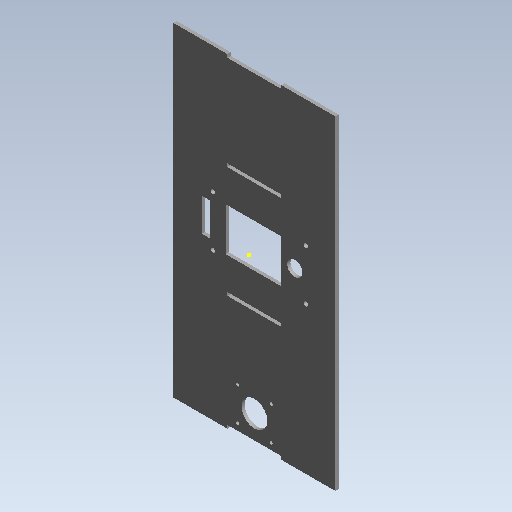
# Autodesk Inventor part: MuurL
Saved by Autodesk Inventor 2020 (Build 240168000, 168)
## iProperties
Part Number: MuurL
Material: Generic
Document SubType Name: Modeling
Designer: SBBA
Appearance: Default
Mass: 124.389 g
Surface Area: 879.905 cm^2
Volume: 124.389 cm^3
Density: 1 g/cm^3
Author: SBBA
Autodesk Inventor part; units mm, degrees
ref_plane "YZ Plane" through (0, 0, 0) normal (1, 0, 0) x (0, 1, 0)
ref_plane "XZ Plane" through (0, 0, 0) normal (0, 1, 0) x (-1, 0, 0)
ref_plane "XY Plane" through (0, 0, 0) normal (0, 0, 1) x (1, 0, 0)
sketch "Sketch1" plane through (0, 0, 0) normal (0, 0, 1) x (1, 0, 0)
  line L0 (-70.3712, 150.7033) -> (79.6288, 150.7033)
  line L1 (79.6288, 150.7033) -> (79.6288, -149.2967)
  line L2 (79.6288, -149.2967) -> (-70.3712, -149.2967)
  line L3 (-70.3712, -149.2967) -> (-70.3712, 150.7033)
  point P0 (0, 0)
  constraints: 8 end point, 2 parallel, 1 horizontal, 1 perpendicular
extrude "Extrusion1" add sketch "Sketch1" along normal blind 3
sketch "Sketch2" plane through (0, 0, 3) normal (0, 0, 1) x (1, 0, 0)
  line L0 (-70.3712, 150.7033) -> (-70.3712, -149.2967) projected
  line L1 (-70.3712, 271.0495) -> (-120.3712, 271.0495)
  line L2 (-20.3712, 147.7184) -> (-20.3712, 150.7184)
  line L3 (-20.3712, 147.7184) -> (29.6288, 147.7184)
  line L4 (29.6288, 147.7184) -> (29.6288, 150.7184)
  line L5 (-20.3712, 150.7184) -> (29.6288, 150.7184)
  line L6 (79.6288, 150.7033) -> (-70.3712, 150.7033) projected
  point P0 (0, 0)
  dimension "d9" = 50
  constraints: 10 end point, 2 horizontal, 2 vertical, 1 parallel, 1 point on line
  measures "d9" distance of L1.start L1.end
extrude "Extrusion2" cut sketch "Sketch2" against normal blind 3
sketch "Sketch3" plane through (0, 0, 3) normal (0, 0, 1) x (1, 0, 0)
  line L0 (-20.3712, 150.7033) -> (-20.3712, 147.7184) projected
  line L1 (-20.3712, -149.2722) -> (29.6288, -149.2967)
  line L2 (79.6288, -149.2967) -> (-70.3712, -149.2967) projected
  line L3 (-20.3712, -149.2722) -> (-20.3712, -146.2722)
  line L4 (-20.3712, -146.2722) -> (29.6288, -146.2967)
  line L5 (29.6288, -146.2967) -> (29.6288, -149.2967)
  point P0 (0, 0)
  constraints: 8 end point, 1 point on line, 1 vertical
extrude "Extrusion3" cut sketch "Sketch3" against normal blind 3
sketch "Sketch4" plane through (0, 0, 3) normal (0, 0, 1) x (1, 0, 0)
  line L0 (29.6288, -46.2722) -> (-20.3712, -46.2722)
  line L1 (-20.3712, -46.2722) -> (29.6288, -46.2722)
  line L2 (29.6288, -46.2722) -> (29.6288, -43.6172)
  line L3 (29.6288, -43.6172) -> (-20.3712, -43.6172)
  line L4 (-20.3712, -43.6172) -> (-20.3712, -46.2722)
  point P0 (0, 0)
  constraints: 10 end point, 2 parallel, 1 horizontal, 1 perpendicular
extrude "Extrusion4" add sketch "Sketch4" against normal blind 3
sketch "Sketch5" plane through (0, 0, 3) normal (0, 0, 1) x (1, 0, 0)
  line L0 (-20.3712, -42.9205) -> (29.6288, -42.9205)
  line L1 (29.6288, -42.9205) -> (29.6288, -39.9205)
  line L2 (29.6288, -39.9205) -> (-20.3712, -39.9205)
  line L3 (-20.3712, -39.9205) -> (-20.3712, -42.9205)
  point P0 (0, 0)
  point P1 (-20.3712, -146.2722)
  point P2 (29.6288, -146.2967)
  constraints: 8 end point, 2 parallel, 1 horizontal, 1 perpendicular
extrude "Extrusion5" cut sketch "Sketch5" against normal blind 3
sketch "Sketch6" plane through (0, 0, 3) normal (0, 0, 1) x (1, 0, 0)
  line L0 (29.6288, -39.9205) -> (-20.3712, -39.9205) projected
  line L1 (-20.3712, 60.1524) -> (29.6288, 60.1524)
  line L2 (29.6288, 60.1524) -> (29.6288, 63.1524)
  line L3 (29.6288, 63.1524) -> (-20.3712, 63.1524)
  line L4 (-20.3712, 63.1524) -> (-20.3712, 60.1524)
  point P0 (0, 0)
  constraints: 8 end point, 2 parallel, 1 horizontal, 1 perpendicular
extrude "Extrusion6" cut sketch "Sketch6" against normal blind 3
sketch "Sketch7" plane through (0, 0, 3) normal (0, 0, 1) x (1, 0, 0)
  line L0 (29.6288, -149.2967) -> (-70.3712, -149.2967) projected
  line L1 (-70.3712, -149.2967) -> (-70.3712, 150.7033) projected
  circle A0 centre (4.6288, -99.2967) radius 12
  point P0 (0, 0)
  constraints: 1 centre point
extrude "Extrusion7" cut sketch "Sketch7" against normal blind 3
sketch "Sketch8" plane through (0, 0, 3) normal (0, 0, 1) x (1, 0, 0)
  circle A0 centre (4.6288, -99.2967) radius 12 projected
  circle A1 centre (20.6853, -83.2968) radius 1.5
  circle A2 centre (-11.3147, -83.2968) radius 1.5
  circle A3 centre (-11.3712, -115.2967) radius 1.5
  circle A4 centre (20.6288, -115.2967) radius 1.5
  point P0 (0, 0)
  constraints: 4 centre point
extrude "Extrusion8" cut sketch "Sketch8" against normal blind 3 contours A1 | A2 | A3 | A4
sketch "Sketch9" plane through (0, 0, 3) normal (0, 0, 1) x (1, 0, 0)
  point P0 (0, 0)
sketch "Sketch11" plane through (0, 0, 3) normal (0, 0, 1) x (1, 0, 0)
  line L0 (-70.3712, 150.7033) -> (-70.3712, -149.2967) projected
  line L1 (79.6288, -149.2967) -> (79.6288, 150.7033) projected
  line L2 (29.6288, 60.1524) -> (-20.3712, 60.1524) projected
  line L3 (-20.3712, -39.9205) -> (29.6288, -39.9205) projected
  circle A0 centre (52.2007, 33.6284) radius 2
  circle A1 centre (52.2018, -13.1716) radius 2
  circle A2 centre (-33.7993, 33.6284) radius 2
  circle A3 centre (-33.7993, -13.1716) radius 2
  line L4 (-43.8689, 25.3776) -> (-36.8689, 25.3776)
  line L5 (-36.8689, 25.3776) -> (-36.8689, -5.0217)
  line L6 (-36.8689, -5.0217) -> (-43.8689, -5.0217)
  line L7 (-43.8689, -5.0217) -> (-43.8689, 25.3776)
  circle A4 centre (41.9518, 10.2284) radius 7
  line L8 (29.0018, -10.3751) -> (-21.9982, -10.3751)
  line L9 (-21.9982, -10.3751) -> (-21.9982, 29.6249)
  line L10 (-21.9982, 29.6249) -> (29.0018, 29.6249)
  line L11 (29.0018, 29.6249) -> (29.0018, -10.3751)
  point P0 (0, 0)
  constraints: 16 end point, 5 centre point, 4 parallel, 2 horizontal, 2 perpendicular
extrude "Extrusion9" cut sketch "Sketch11" against normal blind 30
sketch "Sketch12" plane through (29.6288, -149.2967, 3) normal (0.0005, 1, 0) x (1, -0.0005, 0)
  line L0 (-100, 0) -> (0, 0) projected
  line L1 (-50.0015, 3) -> (0, 3)
  line L2 (0, 3) -> (0, 0)
  line L3 (0, 0) -> (-50.0015, 0)
  line L4 (-50.0015, 0) -> (-50.0015, 3)
  point P0 (-29.7019, 3)
  constraints: 8 end point, 2 parallel, 1 horizontal, 1 perpendicular
extrude "Extrusion10" cut sketch "Sketch12" against normal blind 10
sketch "Sketch13" plane through (0, 0, 3) normal (0, 0, 1) x (1, 0, 0)
  line L0 (29.6288, -146.2967) -> (-20.3712, -146.2722) projected
  circle A0 centre (-11.3147, -83.2968) radius 1.5 projected
  circle A1 centre (-11.3712, -115.2967) radius 1.5 projected
  line L1 (-11.3712, -115.2967) -> (-11.3147, -83.2968)
  circle A2 centre (20.6853, -83.2968) radius 1.5 projected
  line L2 (20.6853, -83.2968) -> (-11.3147, -83.2968)
  line L3 (20.6853, -115.2967) -> (20.6853, -83.2968)
  line L4 (20.6853, -115.2967) -> (-11.3712, -115.2967)
  circle A3 centre (4.6288, -99.2967) radius 12 projected
  line L5 (4.6288, -146.2844) -> (4.6288, -131.2844)
  circle A4 centre (-11.3147, -83.2968) radius 1.5
  circle A5 centre (20.6853, -83.2968) radius 1.5
  circle A6 centre (20.6853, -115.2967) radius 1.455
  circle A7 centre (-11.3712, -115.2967) radius 1.5
  point P0 (0, 0)
  dimension "d107" = 15
  dimension "d108" = 32.0565
  dimension "d109" = 31.9999
  constraints: 10 end point, 4 centre point, 4 coincident, 3 concentric, 2 perpendicular, 1 horizontal, 1 midpoint, 1 vertical
  measures "d107" distance of L5.start L5.end
  measures "d108" distance of L3.start L1.start
  measures "d109" distance of L3.start L2.start
extrude "Extrusion11" add sketch "Sketch13" against normal blind 3 contours L2 L1 A0 | A0 L1 L2 | L2 L3 A2 | A2 L3 L2 | L1 L4 A1 | A1 L4 L1 | A6 L4 L3 | L3 L4 A6
sketch "Sketch14" plane through (0, 0, 3) normal (0, 0, 1) x (1, 0, 0)
  arc A0 (21.8331, -114.4024) -> (21.8331, -116.1909) centre (20.6288, -115.2967) ccw projected
  circle A1 centre (20.6288, -115.2967) radius 2.2964
  point P0 (0, 0)
  constraints: 1 centre point, 1 coincident
extrude "Extrusion12" cut sketch "Sketch14" against normal blind 3
sketch "Sketch15" plane through (0, 0, 3) normal (0, 0, 1) x (1, 0, 0)
  line L0 (17.3499, -111.5348) -> (24.4453, -111.5348)
  line L1 (24.4453, -111.5348) -> (24.4453, -120.5742)
  line L2 (24.4453, -120.5742) -> (17.3499, -120.5742)
  line L3 (17.3499, -120.5742) -> (17.3499, -111.5348)
  point P0 (0, 0)
  constraints: 8 end point, 2 parallel, 1 horizontal, 1 perpendicular
extrude "Extrusion13" cut sketch "Sketch15" against normal blind 3
sketch "Sketch16" plane through (0, 0, 3) normal (0, 0, 1) x (1, 0, 0)
  line L0 (17.3499, -111.5348) -> (24.4453, -111.5348) projected
  line L1 (24.4453, -120.5742) -> (17.3499, -120.5742) projected
  line L2 (17.3499, -111.5348) -> (24.4453, -111.5348)
  line L3 (24.4453, -111.5348) -> (24.4453, -120.5742)
  line L4 (24.4453, -120.5742) -> (17.3499, -120.5742)
  line L5 (17.3499, -120.5742) -> (17.3499, -111.5348)
  point P0 (0, 0)
  constraints: 8 end point, 2 parallel, 1 horizontal, 1 perpendicular
extrude "Extrusion14" add sketch "Sketch16" against normal blind 3
sketch "Sketch17" plane through (0, 0, 3) normal (0, 0, 1) x (1, 0, 0)
  circle A0 centre (4.6288, -99.2967) radius 12 projected
  circle A1 centre (4.6288, -99.2967) radius 12
  point P0 (0, 0)
  constraints: 1 centre point, 1 coincident
extrude "Extrusion15" add sketch "Sketch17" against normal blind 3
sketch "Sketch18" plane through (0, 0, 3) normal (0, 0, 1) x (1, 0, 0)
  line L0 (29.6288, -146.2967) -> (-20.3712, -146.2722) projected
  circle A0 centre (-10.8712, -109.2844) radius 1.5
  circle A1 centre (20.1288, -109.2844) radius 1.5
  circle A2 centre (20.1288, -140.2844) radius 1.5
  circle A3 centre (-10.8712, -140.2844) radius 1.5
  circle A4 centre (4.6288, -124.7844) radius 12
  point P0 (0, 0)
  constraints: 5 centre point
extrude "Extrusion16" cut sketch "Sketch18" against normal blind 35.75
sketch "Sketch19" plane through (0, 0, 3) normal (0, 0, 1) x (1, 0, 0)
  point P0 (0, 0)
body "Solid1"
